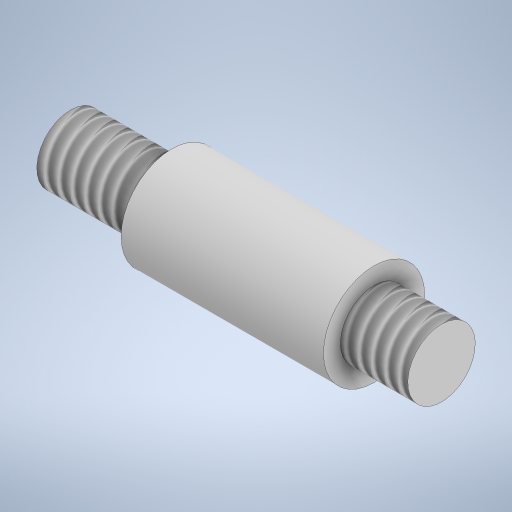
# Autodesk Inventor part: Hudson 1-64
Saved by Autodesk Inventor 2024.2 (Build 282272000, 272)
## iProperties
Created: 2024-10-09
Part Number: Hudson 1-64
Material: Genérico
Document SubType Name: Modeling
Designer: Monica Mora
Density: 1 g/cm^3
Appearance: Valor por defecto
Author: Monica Mora
Autodesk Inventor part; units mm, degrees
ref_plane "YZ Plane" through (0, 0, 0) normal (1, 0, 0) x (0, 1, 0)
ref_plane "XZ Plane" through (0, 0, 0) normal (0, 1, 0) x (-1, 0, 0)
ref_plane "XY Plane" through (0, 0, 0) normal (0, 0, 1) x (1, 0, 0)
sketch "Boceto1" plane through (0, 0, 0) normal (0, 0, 1) x (1, 0, 0)
  line L0 (0, 0) -> (-11, 0)
  line L1 (0, 0) -> (-11, 0)
  line L2 (-11, 0) -> (-11, 1)
  line L3 (0, 1) -> (0, 0)
  line L4 (-8, 0) -> (-2, 0)
  line L5 (-2, 0) -> (-2, 1.5)
  line L6 (-2, 1.5) -> (-8, 1.5)
  line L7 (-8, 1.5) -> (-8, 0)
  line L8 (-11, 1) -> (-8, 1)
  line L9 (-2, 1) -> (0, 1)
  dimension "d1" = 2
  dimension "d2" = 2
  dimension "d3" = 3
  dimension "d4" = 3
  dimension "d5" = 2
  dimension "d6" = 6
  dimension "d7" = 11
  constraints: 20 end point, 5 parallel, 3 horizontal, 3 point on line, 2 perpendicular
  measures "d1" diameter of L9 L0
  measures "d2" distance of L9.start L3.start
  measures "d3" diameter of L6 L0
  measures "d4" distance of L2.end L8.end
  measures "d5" diameter of L8 L0
  measures "d6" distance of L5.end L6.end
  measures "d7" distance of L0.start L0.end
revolve "Revolución1" add sketch "Boceto1" angle 360 about axis through (0, 0, 0) along (-1, 0, 0)
thread "Rosca1" size "M2x0.4" class "6g" standard "ANSI Metric M Profile" length 7
thread "Rosca2" size "M2x0.4" class "6g" standard "ANSI Metric M Profile" length 7
